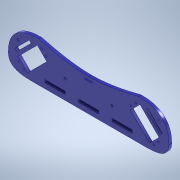
# Autodesk Inventor part: torso side
Saved by Autodesk Inventor 2020.3 (Build 243373000, 373)
## iProperties
Created: 2020-08-06
Part Number: torso side
Material: Generic
Document SubType Name: Modeling
Designer: aditk
Density: 1 g/cm^3
Appearance: Smooth - Navy
Author: aditk
Autodesk Inventor part; units mm, degrees
ref_plane "YZ Plane" through (0, 0, 0) normal (1, 0, 0) x (0, 1, 0)
ref_plane "XZ Plane" through (0, 0, 0) normal (0, 1, 0) x (-1, 0, 0)
ref_plane "XY Plane" through (0, 0, 0) normal (0, 0, 1) x (1, 0, 0)
sketch "Sketch1" plane through (0, 0, 0) normal (0, 0, 1) x (1, 0, 0)
  line L0 (-120, -30) -> (120, -30)
  line L1 (120, -30) -> (120, 30)
  line L2 (120, 30) -> (-120, 30)
  line L3 (-120, 30) -> (-120, -30)
  line L4 (-35.039301, -18.015899) -> (-65.039301, -18.015899)
  line L5 (-65.039301, -18.015899) -> (-65.039301, -22.015899)
  line L6 (-35.039301, -22.015899) -> (-65.039301, -22.015899)
  line L7 (-35.039301, -18.015899) -> (-35.039301, -22.015899)
  line L8 (-35.039301, -18.015899) -> (-35.039301, -22.015899)
  line L9 (-15.039301, -18.015899) -> (-15.039301, -22.015899)
  line L10 (14.960699, -18.015899) -> (-15.039301, -18.015899)
  line L11 (-15.039301, -18.015899) -> (-15.039301, -22.015899)
  line L12 (14.960699, -22.015899) -> (-15.039301, -22.015899)
  line L13 (14.960699, -18.015899) -> (14.960699, -22.015899)
  line L14 (14.960699, -18.015899) -> (14.960699, -22.015899)
  line L15 (34.960699, -18.015899) -> (34.960699, -22.015899)
  line L16 (64.960699, -18.015899) -> (34.960699, -18.015899)
  line L17 (34.960699, -18.015899) -> (34.960699, -22.015899)
  line L18 (64.960699, -22.015899) -> (34.960699, -22.015899)
  line L19 (64.960699, -18.015899) -> (64.960699, -22.015899)
  point P0 (0, 0)
  point P1 (-0.039301, -18.015899)
  constraints: 40 end point, 2 parallel, 1 horizontal, 1 perpendicular
extrude "Extrusion1" add sketch "Sketch1" along normal blind 4
sketch "Sketch2" plane through (0, 0, 4) normal (0, 0, 1) x (1, 0, 0)
  line L0 (-120, 30) -> (-120, -30)
  line L1 (-110, 0) -> (-88.786797, 21.213203)
  line L2 (-88.786797, 21.213203) -> (-85.958369, 18.384776)
  line L3 (-85.958369, 18.384776) -> (-107.171573, -2.828427)
  line L4 (-107.171573, -2.828427) -> (-110, 0)
  line L5 (120, 30) -> (-120, 30)
  line L6 (110, 0) -> (88.786797, 21.213203)
  line L7 (88.786797, 21.213203) -> (85.958369, 18.384776)
  line L8 (85.958369, 18.384776) -> (107.171573, -2.828427)
  line L9 (107.171573, -2.828427) -> (110, 0)
  point P0 (0, 0)
  constraints: 16 end point, 3 perpendicular
extrude "Extrusion2" cut sketch "Sketch2" against normal through all
sketch "Sketch3" plane through (0, 0, 4) normal (0, 0, 1) x (1, 0, 0)
  line L0 (110, 0) -> (107.171573, -2.828427)
  line L1 (107.171573, -2.828427) -> (85.958369, 18.384776)
  line L2 (85.958369, 18.384776) -> (88.786797, 21.213203)
  line L3 (88.786797, 21.213203) -> (110, 0)
  line L4 (-88.786797, 21.213203) -> (-85.958369, 18.384776)
  line L5 (-85.958369, 18.384776) -> (-107.171573, -2.828427)
  line L6 (-107.171573, -2.828427) -> (-110, 0)
  line L7 (-110, 0) -> (-88.786797, 21.213203)
  line L8 (120, -30) -> (120, 30)
  line L9 (120, 30) -> (-120, 30)
  line L10 (-120, 30) -> (-120, -30)
  line L11 (-120, -30) -> (120, -30)
  line L12 (-65.039301, -18.015899) -> (-35.039301, -18.015899)
  line L13 (-35.039301, -18.015899) -> (-35.039301, -22.015899)
  line L14 (-35.039301, -22.015899) -> (-65.039301, -22.015899)
  line L15 (-65.039301, -22.015899) -> (-65.039301, -18.015899)
  line L16 (64.960699, -22.015899) -> (34.960699, -22.015899)
  line L17 (34.960699, -22.015899) -> (34.960699, -18.015899)
  line L18 (34.960699, -18.015899) -> (64.960699, -18.015899)
  line L19 (64.960699, -18.015899) -> (64.960699, -22.015899)
  line L20 (-15.039301, -18.015899) -> (14.960699, -18.015899)
  line L21 (14.960699, -18.015899) -> (14.960699, -22.015899)
  line L22 (14.960699, -22.015899) -> (-15.039301, -22.015899)
  line L23 (-15.039301, -22.015899) -> (-15.039301, -18.015899)
  line L24 (120, 30) -> (-120, 30)
  line L25 (-120, 30) -> (-120, -30)
  line L26 (-120, -10) -> (-120, 30) construction
  line L27 (-120, 30) -> (-74.343146, 30) construction
  spline S0 degree 2 poles (-120, -10) (-120, 30) (-74.343146, 30) knots 1 1 1 2 2 2
  line L28 (-74.343146, 30) -> (-30.816047, 18.384776) construction
  line L29 (-30.816047, 18.384776) -> (0, 18.384776) construction
  spline S1 degree 2 poles (-74.343146, 30) (-30.816047, 18.384776) (0, 18.384776) knots 1 1 1 2 2 2
  line L30 (-120, -10) -> (-120, -23.511577) construction
  line L31 (-120, -30) -> (120, -30)
  line L32 (-120, -23.511577) -> (-110, -30) construction
  line L33 (-110, -30) -> (-95.168595, -30) construction
  line L34 (-95.168595, -30) -> (-80, -30) construction
  spline S2 degree 4 poles (-120, -10) (-120, -23.511577) (-110, -30) (-95.168595, -30) (-80, -30) knots 1 1 1 1 1 2 2 2 2 2
  line L35 (-80, -30) -> (-120, -30)
  line L36 (-120, -10) -> (-120, 30)
  line L37 (-74.343146, 30) -> (0, 30)
  line L38 (-120, -30) -> (-120, -10)
  line L39 (-120, 30) -> (-74.343146, 30)
  line L40 (0, 30) -> (0, -30)
  line L41 (-120, 30) -> (120, 30)
  line L42 (120, 30) -> (120, -30)
  line L43 (-120, 30) -> (120, 30)
  line L44 (120, 30) -> (120, -30)
  line L45 (120, -10) -> (120, 30) construction
  line L46 (120, 30) -> (74.343146, 30) construction
  spline S3 degree 2 poles (120, -10) (120, 30) (74.343146, 30) knots 1 1 1 2 2 2
  line L47 (74.343146, 30) -> (30.816047, 18.384776) construction
  line L48 (30.816047, 18.384776) -> (0, 18.384776) construction
  spline S4 degree 2 poles (74.343146, 30) (30.816047, 18.384776) (0, 18.384776) knots 1 1 1 2 2 2
  line L49 (120, -10) -> (120, -23.511577) construction
  line L50 (120, -23.511577) -> (110, -30) construction
  line L51 (110, -30) -> (95.168595, -30) construction
  line L52 (95.168595, -30) -> (80, -30) construction
  spline S5 degree 4 poles (120, -10) (120, -23.511577) (110, -30) (95.168595, -30) (80, -30) knots 1 1 1 1 1 2 2 2 2 2
  line L53 (80, -30) -> (120, -30)
  line L54 (74.343146, 30) -> (0, 30)
  line L55 (120, -30) -> (120, -10)
  line L56 (120, 30) -> (74.343146, 30)
  point P0 (0, 0)
  point P1 (80.002249, -30)
  point P2 (-80.002249, -30)
  constraints: 28 end point, 12 symmetric about line, 11 point on line, 4 coincident, 3 collinear, 2 midpoint, 2 perpendicular, 1 parallel, 18 other
sketch "Sketch3 outline for Extrusion3" plane through (0, 0, 4) normal (0, 0, 1) x (1, 0, 0)
  spline S0 degree 2 poles (120, -10) (120, 30) (74.343146, 30) knots 0 0 0 1 1 1
  line L0 (120, 30) -> (74.343146, 30)
  line L1 (120, -10) -> (120, 30)
  line L2 (74.343146, 30) -> (-74.343146, 30)
  spline S1 degree 2 poles (74.343146, 30) (30.816047, 18.384776) (0, 18.384776) knots 0 0 0 1 1 1
  spline S2 degree 2 poles (-74.343146, 30) (-30.816047, 18.384776) (0, 18.384776) knots 0 0 0 1 1 1
  spline S3 degree 4 poles (120, -10) (120, -23.511076) (110.000741, -29.999519) (95.170245, -30) (80.002249, -30) knots 0 0 0 0 0 1 1 1 1 1
  line L3 (120, -30) -> (120, -10)
  line L4 (80.002249, -30) -> (120, -30)
  spline S4 degree 2 poles (-120, -10) (-120, 30) (-74.343146, 30) knots 0 0 0 1 1 1
  line L5 (-120, 30) -> (-120, -10)
  line L6 (-74.343146, 30) -> (-120, 30)
  spline S5 degree 4 poles (-120, -10) (-120, -23.511076) (-110.000741, -29.999519) (-95.170245, -30) (-80.002249, -30) knots 0 0 0 0 0 1 1 1 1 1
  line L7 (-120, -30) -> (-80.002249, -30)
  line L8 (-120, -10) -> (-120, -30)
extrude "Extrusion3" cut sketch "Sketch3 outline for Extrusion3" against normal through all
sketch "Sketch4" plane through (0, 0, 4) normal (0, 0, 1) x (1, 0, 0)
  line L0 (-76.678629, -7.832244) -> (-62.465783, 6.380603)
  line L1 (-62.465783, 6.380603) -> (-76.678629, 20.593449)
  line L2 (-76.678629, 20.593449) -> (-105.104321, -7.832244)
  line L3 (-105.104321, -7.832244) -> (-90.891475, -22.04509)
  line L4 (-90.891475, -22.04509) -> (-76.678629, -7.832244)
  line L5 (-76.678629, -7.832244) -> (-57.233192, 11.613193)
  line L6 (-57.233192, 11.613193) -> (-71.446039, 25.826039)
  line L7 (-71.446039, 25.826039) -> (-76.678629, 20.593449)
  line L8 (-105.104321, -7.832244) -> (-110.336912, -13.064834)
  line L9 (-110.336912, -13.064834) -> (-96.124065, -27.27768)
  line L10 (-96.124065, -27.27768) -> (-90.891475, -22.04509)
  circle A0 centre (-70.440384, 19.587794) radius 1.1
  circle A1 centre (-63.471437, 12.618848) radius 1.1
  circle A2 centre (-104.098667, -14.070488) radius 1.1
  circle A3 centre (-97.12972, -21.039435) radius 1.1
  line L11 (76.678629, -7.832244) -> (62.465783, 6.380603)
  line L12 (62.465783, 6.380603) -> (76.678629, 20.593449)
  line L13 (76.678629, 20.593449) -> (105.104321, -7.832244)
  line L14 (105.104321, -7.832244) -> (90.891475, -22.04509)
  line L15 (90.891475, -22.04509) -> (76.678629, -7.832244)
  line L16 (76.678629, -7.832244) -> (57.233192, 11.613193)
  line L17 (57.233192, 11.613193) -> (71.446039, 25.826039)
  line L18 (71.446039, 25.826039) -> (76.678629, 20.593449)
  line L19 (105.104321, -7.832244) -> (110.336912, -13.064834)
  line L20 (110.336912, -13.064834) -> (96.124065, -27.27768)
  line L21 (96.124065, -27.27768) -> (90.891475, -22.04509)
  circle A4 centre (70.440384, 19.587794) radius 1.1
  circle A5 centre (63.471437, 12.618848) radius 1.1
  circle A6 centre (97.12972, -21.039435) radius 1.1
  circle A7 centre (104.098667, -14.070488) radius 1.1
  point P0 (0, 0)
  point P1 (107.171573, -2.828427)
  point P2 (85.958369, 18.384776)
  constraints: 44 end point, 8 centre point, 8 perpendicular, 6 point on line
extrude "Extrusion4" cut sketch "Sketch4" against normal through all contours L4 L3 L2 L1 L0 | A0 | A1 | A2 | A3 | L11 L12 L13 L14 L15 | A4 | A5 | A6 | A7
sketch "Sketch5" plane through (0, 0, 0) normal (0, 0, -1) x (-1, 0, 0)
  circle A0 centre (97.12972, -21.039435) radius 1.1
  circle A1 centre (-70.440384, 19.587794) radius 1.1
  line L0 (-105.104321, -7.832244) -> (-76.678629, 20.593449)
  line L1 (-76.678629, 20.593449) -> (-62.465783, 6.380603)
  line L2 (-62.465783, 6.380603) -> (-90.891475, -22.04509)
  line L3 (-90.891475, -22.04509) -> (-105.104321, -7.832244)
  circle A2 centre (-63.471437, 12.618848) radius 1.1
  circle A3 centre (104.098667, -14.070488) radius 1.1
  circle A4 centre (70.440384, 19.587794) radius 1.1
  circle A5 centre (-97.12972, -21.039435) radius 1.1
  circle A6 centre (-104.098667, -14.070488) radius 1.1
  circle A7 centre (63.471437, 12.618848) radius 1.1
  line L4 (62.465783, 6.380603) -> (76.678629, 20.593449)
  line L5 (76.678629, 20.593449) -> (105.104321, -7.832244)
  line L6 (105.104321, -7.832244) -> (90.891475, -22.04509)
  line L7 (90.891475, -22.04509) -> (62.465783, 6.380603)
  line L8 (15.039301, -18.015899) -> (-14.960699, -18.015899)
  line L9 (15.039301, -22.015899) -> (15.039301, -18.015899)
  line L10 (-14.960699, -22.015899) -> (15.039301, -22.015899)
  line L11 (-14.960699, -18.015899) -> (-14.960699, -22.015899)
  line L12 (-64.960699, -22.015899) -> (-34.960699, -22.015899)
  line L13 (-64.960699, -18.015899) -> (-64.960699, -22.015899)
  line L14 (-34.960699, -18.015899) -> (-64.960699, -18.015899)
  line L15 (-34.960699, -22.015899) -> (-34.960699, -18.015899)
  line L16 (65.039301, -18.015899) -> (35.039301, -18.015899)
  line L17 (65.039301, -22.015899) -> (65.039301, -18.015899)
  line L18 (35.039301, -22.015899) -> (65.039301, -22.015899)
  line L19 (35.039301, -18.015899) -> (35.039301, -22.015899)
  line L20 (85.958369, 18.384776) -> (88.786797, 21.213203)
  line L21 (88.786797, 21.213203) -> (110, 0)
  line L22 (110, 0) -> (107.171573, -2.828427)
  line L23 (107.171573, -2.828427) -> (85.958369, 18.384776)
  line L24 (-107.171573, -2.828427) -> (-110, 0)
  line L25 (-110, 0) -> (-88.786797, 21.213203)
  line L26 (-88.786797, 21.213203) -> (-85.958369, 18.384776)
  line L27 (-85.958369, 18.384776) -> (-107.171573, -2.828427)
  line L28 (80.002249, -30) -> (-80.002249, -30)
  circle A8 centre (-105.198667, 13.487026) radius 1.5
  circle A9 centre (-34.960699, 13.487026) radius 1.5
  circle A10 centre (105.198667, 13.487026) radius 1.5
  circle A11 centre (34.960699, 13.487026) radius 1.5
  point P0 (0, 0)
  constraints: 4 centre point, 6 other
extrude "Extrusion5" cut sketch "Sketch5" against normal blind 10 contours A8 | A9 | A10 | A11
move faces "Move1" translate (0, -15, 0) faces at (35.021098, 11.988242, 2.666667)
move faces "Move2" translate (0, -15, 0) faces at (-34.9003, 11.988242, 2.666667)
sketch "Sketch6" plane through (0, 0, 4) normal (0, 0, 1) x (1, 0, 0)
  spline S0 degree 3 poles (-74.343146, 30) (-35.666012, 20.499455) (-23.035589, 18.96661) (0, 18.384776) knots 0 0 0 0 1 1 1 1
  spline S1 degree 2 poles (-74.343146, 30) (0, -13.230447) (74.343146, 30) knots 0 0 0 1 1 1
  spline S2 degree 3 poles (0, 18.384776) (23.036688, 18.965649) (35.666908, 20.489849) (74.343146, 30) knots 0 0 0 0 1 1 1 1
  line L0 (0, 18.384776) -> (0, 8.384776)
  line L1 (-5, 13.384776) -> (5, 13.384776) construction
  line L2 (-5, 12.384776) -> (5, 12.384776)
  line L3 (5, 14.384776) -> (-5, 14.384776)
  arc A0 (-5, 14.384776) -> (-5, 12.384776) centre (-5, 13.384776) ccw
  arc A1 (5, 12.384776) -> (5, 14.384776) centre (5, 13.384776) ccw
  circle A2 centre (-34.960699, -1.512974) radius 1.5
  circle A3 centre (34.960699, -1.512974) radius 1.5
  circle A4 centre (-105.198667, 13.487026) radius 1.5
  circle A5 centre (105.198667, 13.487026) radius 1.5
  circle A6 centre (-97.12972, -21.039435) radius 1.1
  circle A7 centre (70.440384, 19.587794) radius 1.1
  line L4 (76.678629, 20.593449) -> (105.104321, -7.832244)
  line L5 (105.104321, -7.832244) -> (90.891475, -22.04509)
  line L6 (90.891475, -22.04509) -> (62.465783, 6.380603)
  line L7 (62.465783, 6.380603) -> (76.678629, 20.593449)
  circle A8 centre (63.471437, 12.618848) radius 1.1
  circle A9 centre (-104.098667, -14.070488) radius 1.1
  circle A10 centre (-70.440384, 19.587794) radius 1.1
  circle A11 centre (97.12972, -21.039435) radius 1.1
  circle A12 centre (104.098667, -14.070488) radius 1.1
  circle A13 centre (-63.471437, 12.618848) radius 1.1
  line L8 (-76.678629, 20.593449) -> (-62.465783, 6.380603)
  line L9 (-62.465783, 6.380603) -> (-90.891475, -22.04509)
  line L10 (-90.891475, -22.04509) -> (-105.104321, -7.832244)
  line L11 (-105.104321, -7.832244) -> (-76.678629, 20.593449)
  line L12 (-80.002249, -30) -> (80.002249, -30)
  line L13 (110, 0) -> (107.171573, -2.828427)
  line L14 (107.171573, -2.828427) -> (85.958369, 18.384776)
  line L15 (85.958369, 18.384776) -> (88.786797, 21.213203)
  line L16 (88.786797, 21.213203) -> (110, 0)
  line L17 (-88.786797, 21.213203) -> (-85.958369, 18.384776)
  line L18 (-85.958369, 18.384776) -> (-107.171573, -2.828427)
  line L19 (-107.171573, -2.828427) -> (-110, 0)
  line L20 (-110, 0) -> (-88.786797, 21.213203)
  line L21 (-65.039301, -18.015899) -> (-35.039301, -18.015899)
  line L22 (-35.039301, -18.015899) -> (-35.039301, -22.015899)
  line L23 (-35.039301, -22.015899) -> (-65.039301, -22.015899)
  line L24 (-65.039301, -22.015899) -> (-65.039301, -18.015899)
  line L25 (64.960699, -22.015899) -> (34.960699, -22.015899)
  line L26 (34.960699, -22.015899) -> (34.960699, -18.015899)
  line L27 (34.960699, -18.015899) -> (64.960699, -18.015899)
  line L28 (64.960699, -18.015899) -> (64.960699, -22.015899)
  line L29 (-15.039301, -18.015899) -> (14.960699, -18.015899)
  line L30 (14.960699, -18.015899) -> (14.960699, -22.015899)
  line L31 (14.960699, -22.015899) -> (-15.039301, -22.015899)
  line L32 (-15.039301, -22.015899) -> (-15.039301, -18.015899)
  point P0 (0, 0)
  point P1 (0, 0)
  point P2 (0, 13.384776)
  dimension "d31" = 5
  dimension "d32" = 2
  constraints: 10 end point, 4 point on circle, 4 tangent, 2 centre point, 2 midpoint, 1 parallel, 1 perpendicular, 1 vertical, 16 other
  measures "d31" distance of point (0, 13.385) L1.end
  measures "d32" diameter of A1
extrude "Extrusion6" cut sketch "Sketch6" against normal through all contours L3 A1 L2 L0 | L0 L2 A0 L3
body "Solid1"
